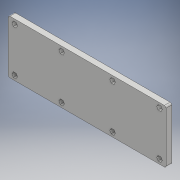
# Autodesk Inventor part: Part1
Saved by Autodesk Inventor 2017 SP1 (Build 210196100, 196)
## iProperties
Created: 2018-02-12
Part Number: Part1
Material: Generic
Document SubType Name: Modeling
Designer: Sung Dz-da
Density: 1 g/cm^3
Appearance: Default
Author: Sung Dz-da
Autodesk Inventor part; units mm, degrees
ref_plane "YZ Plane" through (0, 0, 0) normal (1, 0, 0) x (0, 1, 0)
ref_plane "XZ Plane" through (0, 0, 0) normal (0, 1, 0) x (-1, 0, 0)
ref_plane "XY Plane" through (0, 0, 0) normal (0, 0, 1) x (1, 0, 0)
sketch "Sketch1" plane through (0, 0, 0) normal (0, 1, 0) x (-1, 0, 0)
  line L0 (97.5, -33) -> (-97.5, -33)
  line L1 (-97.5, -33) -> (-97.5, 33)
  line L2 (-97.5, 33) -> (97.5, 33)
  line L3 (97.5, 33) -> (97.5, -33)
  line L4 (97.5, -33) -> (-97.5, 33) construction
  line L5 (-97.5, -33) -> (97.5, 33) construction
  point P0 (0, 0)
  dimension "d0" = 195
  dimension "d1" = 66
  constraints: 12 end point, 2 midpoint, 2 parallel, 1 horizontal, 1 perpendicular
  measures "d0" distance of L1.end L2.end
  measures "d1" distance of L0.end L1.end
extrude "Extrusion1" add sketch "Sketch1" along normal blind 7
fillet "Fillet1" radius 2 4 edges at (-97.5, 3.5, 33) (97.5, 3.5, 33) (97.5, 3.5, -33) (-97.5, 3.5, -33)
sketch "Sketch2" plane through (0, 7, 0) normal (0, 1, 0) x (1, 0, 0)
  line L0 (-32.5, 27.25) -> (-30.5, 27.25) construction
  line L1 (-32.5, 25.65) -> (-30.5, 25.65)
  line L2 (-30.5, 28.85) -> (-32.5, 28.85)
  arc A0 (-32.5, 28.85) -> (-32.5, 25.65) centre (-32.5, 27.25) ccw
  arc A1 (-30.5, 25.65) -> (-30.5, 28.85) centre (-30.5, 27.25) ccw
  circle A2 centre (-89.5, 27.25) radius 1.6
  line L3 (30.5, 27.25) -> (32.5, 27.25) construction
  line L4 (30.5, 25.65) -> (32.5, 25.65)
  line L5 (32.5, 28.85) -> (30.5, 28.85)
  arc A3 (30.5, 28.85) -> (30.5, 25.65) centre (30.5, 27.25) ccw
  arc A4 (32.5, 25.65) -> (32.5, 28.85) centre (32.5, 27.25) ccw
  line L6 (88.5, 27.25) -> (90.5, 27.25) construction
  line L7 (88.5, 25.65) -> (90.5, 25.65)
  line L8 (90.5, 28.85) -> (88.5, 28.85)
  arc A5 (88.5, 28.85) -> (88.5, 25.65) centre (88.5, 27.25) ccw
  arc A6 (90.5, 25.65) -> (90.5, 28.85) centre (90.5, 27.25) ccw
  line L9 (95.5, 33) -> (-95.5, 33) projected
  line L10 (-97.5, 31) -> (-97.5, -31) projected
  line L11 (97.5, -31) -> (97.5, 31) projected
  point P0 (0, 0)
  point P1 (-31.5, 27.25)
  point P2 (31.5, 27.25)
  point P3 (89.5, 27.25)
  dimension "d9" = 1
  dimension "d10" = 3.2
  dimension "d11" = 3.2
  dimension "d12" = 1
  dimension "d13" = 3.2
  dimension "d14" = 1
  dimension "d15" = 3.2
  dimension "d16" = 58
  dimension "d17" = 63
  dimension "d18" = 58
  dimension "d19" = 5.75
  dimension "d21" = 8
  constraints: 24 end point, 12 point on circle, 12 tangent, 7 centre point, 3 horizontal, 3 midpoint, 3 parallel, 2 horizontal alignment, 1 collinear
  measures "d9" distance of point (-31.5, 27.25) L0.end
  measures "d10" diameter of A1
  measures "d11" diameter of A2
  measures "d12" distance of point (31.5, 27.25) L3.end
  measures "d13" diameter of A4
  measures "d14" distance of point (89.5, 27.25) L6.end
  measures "d15" diameter of A6
  measures "d16" distance of point (-31.5, 27.25) A2.centre
  measures "d17" distance of point (31.5, 27.25) point (-31.5, 27.25)
  measures "d18" distance of point (89.5, 27.25) point (31.5, 27.25)
  measures "d19" distance from line of point (-31.5, 27.25) L9
  measures "d21" distance from line of point (89.5, 27.25) L11
extrude "Extrusion2" cut sketch "Sketch2" against normal through all
mirror "Mirror1" about plane through (0, 0, 0) normal (0, 0, 1) of "Extrusion2"
sketch "Sketch3" plane through (0, 0, 0) normal (0, -1, 0) x (1, 0, 0)
  circle A0 centre (-89.5, -27.25) radius 1.6 projected
  line L0 (-87.7679, -24.25) -> (-86.0359, -27.25)
  line L1 (-86.0359, -27.25) -> (-87.7679, -30.25)
  line L2 (-87.7679, -30.25) -> (-91.2321, -30.25)
  line L3 (-91.2321, -30.25) -> (-92.9641, -27.25)
  line L4 (-92.9641, -27.25) -> (-91.2321, -24.25)
  line L5 (-91.2321, -24.25) -> (-87.7679, -24.25)
  point P0 (0, 0)
  dimension "d24" = 3
  constraints: 12 end point, 1 coincident, 1 horizontal, 13 other
  measures "d24" distance from line of point (-89.5, -27.25) L5
extrude "Extrusion3" cut sketch "Sketch3" against normal blind 5
pattern_linear "Rectangular Pattern1" count 2 spacing 58 along (1, 0, 0) of "Extrusion3"
mirror "Mirror2" about plane through (0, 0, 0) normal (0, 0, 1) of "Extrusion3", "Rectangular Pattern1"
mirror "Mirror3" about plane through (0, 0, 0) normal (1, 0, 0) of "Extrusion3", "Rectangular Pattern1", "Mirror2"
body "Solid1"
